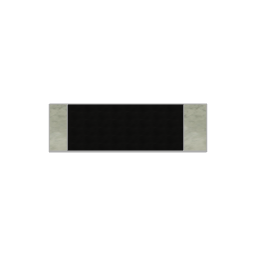
_Curve Fill.cbb05daa-f018-4d11-9b41-78890b19e25e (Autodesk Fusion 360 design; units mm, degrees)
Autodesk Fusion 360 part; units mm, degrees
sketch "sketch 339" plane through (0, 0, -15.1746) normal (0, 0, 1) x (-1, 0, 0)
  line L0 (4684.059, -3219.2162) -> (4253.0067, -3650.2685)
  line L1 (4684.059, -3219.2162) -> (4253.0067, -3650.2685)
  line L2 (4684.059, -3219.2162) -> (4382.4214, -2917.5786)
  line L3 (4684.059, -3219.2162) -> (4382.4214, -2917.5786)
  line L4 (3951.3691, -3348.6309) -> (4382.4214, -2917.5786)
  line L5 (4253.0067, -3650.2685) -> (3951.3691, -3348.6309)
  line L6 (4253.0067, -3650.2685) -> (3951.3691, -3348.6309)
extrude "Extrude1" add sketch "sketch 339" along normal blind 6.35
sketch "sketch 364" plane through (0, 0, -15.1746) normal (0, 0, 1) x (-1, 0, 0)
  line L0 (4450, -2850) -> (4751.6376, -3151.6376)
  line L1 (4382.4214, -2917.5786) -> (4450, -2850)
  line L2 (4684.059, -3219.2162) -> (4382.4214, -2917.5786)
  line L3 (4684.059, -3219.2162) -> (4382.4214, -2917.5786)
  line L4 (4751.6376, -3151.6376) -> (4684.059, -3219.2162)
  line L5 (4166.8953, -3736.38) -> (4253.0067, -3650.2685)
  line L6 (4253.0067, -3650.2685) -> (3951.3691, -3348.6309)
  line L7 (4253.0067, -3650.2685) -> (3951.3691, -3348.6309)
  line L8 (3951.3691, -3348.6309) -> (3865.2576, -3434.7424)
  line L9 (3865.2576, -3434.7424) -> (4166.8953, -3736.38)
extrude "Extrude2" add sketch "sketch 364" along normal blind 6.096
